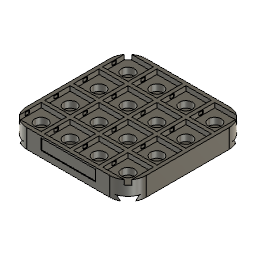
switchbox_choc (Autodesk Fusion 360 design; units mm, degrees)
Autodesk Fusion 360 part; units mm, degrees
sketch "outer_profile" plane through (0, 0, 0) normal (0, 0, 1) x (1, 0, 0)
  line L0 (32.8, 32.8) -> (-32.8, 32.8)
  line L1 (-32.8, 32.8) -> (-32.8, -32.8)
  line L2 (-32.8, -32.8) -> (32.8, -32.8)
  line L3 (32.8, -32.8) -> (32.8, 32.8)
  line L4 (-32.8, -32.8) -> (32.8, 32.8) construction
  dimension "d27" = 65.6
  dimension "d28" = 65.6
  constraint horizontal L0
  constraint horizontal L2
  constraint vertical L1
  constraint vertical L3
  constraint midpoint origin L4
  measures "d27" horizontal distance of L0.start L0.end
  measures "d28" vertical distance of L0.end L1.end
extrude "block" add sketch "outer_profile" along normal blind 10.45
fillet "corner_fillets" radius 10 4 edges at (32.8, -32.8, 5.225) (-32.8, -32.8, 5.225) (-32.8, 32.8, 5.225) (32.8, 32.8, 5.225)
ref_plane "WorkPlane1" through (0, 0, 10.45) normal (0, 0, 1) x (1, 0, 0)
sketch "pocket_seed" plane through (0, 0, 10.45) normal (0, 0, 1) x (1, 0, 0)
  line L0 (-16.9, -16.9) -> (-30.8, -16.9)
  line L1 (-30.8, -16.9) -> (-30.8, -30.8)
  line L2 (-30.8, -30.8) -> (-16.9, -30.8)
  line L3 (-16.9, -30.8) -> (-16.9, -16.9)
  line L4 (-30.8, -30.8) -> (-16.9, -16.9) construction
  dimension "d35" = 13.9
  dimension "d36" = 13.9
  dimension "d58" = 30.8
  dimension "d59" = 30.8
  constraint horizontal L0
  constraint horizontal L2
  constraint vertical L1
  constraint vertical L3
  measures "d35" horizontal distance of L0.start L0.end
  measures "d36" vertical distance of L0.end L1.end
  measures "d58" horizontal distance of origin L1.end
  measures "d59" vertical distance of origin L1.end
extrude "pocket_cut" cut sketch "pocket_seed" against normal blind 2.6
ref_plane "WorkPlane2" through (0, 0, 7.85) normal (0, 0, 1) x (1, 0, 0)
sketch "relief_seed" plane through (0, 0, 7.85) normal (0, 0, 1) x (1, 0, 0)
  circle A0 centre (-23.85, -23.85) radius 3.5
  dimension "d41" = 7
  dimension "d62" = 23.85
  dimension "d63" = 23.85
  measures "d41" diameter of A0
  measures "d62" horizontal distance of origin A0.centre
  measures "d63" vertical distance of origin A0.centre
extrude "relief_cut" cut sketch "relief_seed" against normal blind 3.6
ref_plane "WorkPlane3" through (0, 0, 8.45) normal (0, 0, 1) x (1, 0, 0)
sketch "rib_seed" plane through (0, 0, 8.45) normal (0, 0, 1) x (1, 0, 0)
  line L0 (-30.8, -25.6869) -> (-30.6, -23.85)
  line L1 (-30.6, -23.85) -> (-30.8, -23.2869)
  line L2 (-30.8, -23.2869) -> (-30.8, -25.6869)
  line L3 (-16.9, -24.6706) -> (-17.1, -23.85)
  line L4 (-17.1, -23.85) -> (-16.9, -22.2706)
  line L5 (-16.9, -22.2706) -> (-16.9, -24.6706)
  dimension "d91" = 30.8
  dimension "d92" = 30.6
  dimension "d93" = 2.4
  dimension "d94" = 23.85
  dimension "d95" = 16.9
  dimension "d96" = 17.1
  dimension "d97" = 2.4
  constraint vertical L2
  constraint vertical L5
  constraint horizontal L0.end L3.end
  measures "d91" horizontal distance of origin L0.start
  measures "d92" horizontal distance of origin L0.end
  measures "d93" vertical distance of L0.start L1.end
  measures "d94" vertical distance of origin L0.end
  measures "d95" horizontal distance of origin L3.start
  measures "d96" horizontal distance of origin L3.end
  measures "d97" vertical distance of L3.start L4.end
extrude "snap_ribs" add sketch "rib_seed" along normal blind 1.6
pattern_linear "pocket_grid" count 4 spacing 15.9 along (1, 0, 0) count 4 spacing 15.9 along (0, 1, 0) of "pocket_cut", "relief_cut", "snap_ribs"
sketch "stack_ring" plane through (0, 0, 0) normal (0, 0, 1) x (1, 0, 0)
  line L0 (31.6, 31.6) -> (-31.6, 31.6)
  line L1 (-31.6, 31.6) -> (-31.6, -31.6)
  line L2 (-31.6, -31.6) -> (31.6, -31.6)
  line L3 (31.6, -31.6) -> (31.6, 31.6)
  line L4 (-31.6, -31.6) -> (31.6, 31.6) construction
  dimension "d104" = 63.2
  dimension "d105" = 63.2
  constraint horizontal L0
  constraint horizontal L2
  constraint vertical L1
  constraint vertical L3
  constraint midpoint origin L4
  measures "d104" horizontal distance of L0.start L0.end
  measures "d105" vertical distance of L0.end L1.end
extrude "stack_ring_cut" cut sketch "stack_ring" along normal blind 2.5 draft 15
sketch "label_pocket" plane through (0, -32.8, 0) normal (0, -1, 0) x (1, 0, 0)
  line L0 (-22.8, 10.45) -> (-22.8, 0)
  line L1 (-22.8, 0) -> (22.8, 0)
  line L2 (22.8, 0) -> (22.8, 10.45)
  line L3 (22.8, 10.45) -> (-22.8, 10.45)
  line L4 (15, 9.45) -> (-15, 9.45)
  line L5 (-15, 9.45) -> (-15, 3.5)
  line L6 (-15, 3.5) -> (15, 3.5)
  line L7 (15, 3.5) -> (15, 9.45)
  line L8 (-15, 3.5) -> (15, 9.45) construction
  point P0 (0, 6.475)
  dimension "d123" = 30
  dimension "d124" = 5.95
  dimension "d125" = 6.475
  dimension "d126" = 0
  constraint midpoint L8 P0
  measures "d123" horizontal distance of L4.start L4.end
  measures "d124" vertical distance of L4.end L5.end
  measures "d125" vertical distance of origin P0
  measures "d126" horizontal distance of origin P0
extrude "label_cut" cut sketch "label_pocket" against normal blind 0.4 contours L4 L5 L6 L7
equation "cols = 4 mm" comment "Number of switch columns (2-10)"
equation "rows = 4 mm" comment "Number of switch rows (2-10)"
equation "wall = 2.0 mm" comment "Wall thickness in mm (min 1.75)"
equation "rib_depth = 0.2 mm" comment "Snap tightness in mm: lower is looser, 0.2 default"
equation "corner_fillet = 10 mm" comment "Vertical corner radius in mm"
equation "label_w = 30 mm" comment "Front label width in mm (auto-clamped to fit)"
equation "label_h = 12 mm" comment "Front label height in mm (auto-clamped to fit)"
equation "label_depth = 0.4 mm" comment "Front label recess depth in mm (auto-clamped)"
equation "stack_angle = 75 deg" comment "Stacking ring draft angle in degrees"
equation "pocket_size = 13.9 mm" comment "Switch pocket size (Choc)"
equation "pocket_depth = 2.6 mm" comment "Pocket depth to floor (Choc)"
equation "relief_dia = 7.0 mm" comment "Pin relief diameter"
equation "relief_depth = 3.6 mm" comment "Pin relief depth"
equation "floor_t = 1.75 mm" comment "Floor thickness below relief"
equation "ring_h = 2.5 mm" comment "Stack ring height"
equation "ring_inset = 1.2 mm" comment "Stack ring inset from outer wall"
equation "pitch = pocket_size + wall" comment "Pocket centre-to-centre pitch"
equation "box_x = ( cols / 1 mm ) * pitch + wall" comment "Overall box X"
equation "box_y = ( rows / 1 mm ) * pitch + wall" comment "Overall box Y"
equation "box_h = pocket_depth + relief_depth + floor_t + ring_h" comment "Overall box height"
equation "d27 = box_x"
equation "d28 = box_y"
equation "d29 = box_h"
equation "d32 = corner_fillet"
equation "d33 = box_h"
equation "d35 = pocket_size"
equation "d36 = pocket_size"
equation "d37 = -pocket_depth"
equation "d39 = box_h - pocket_depth"
equation "d41 = relief_dia"
equation "d42 = -relief_depth"
equation "rib_w = 2.4 mm" comment "Snap rib width along the pocket wall"
equation "rib_h = 1.6 mm" comment "Snap rib vertical height"
equation "rib_top_off = 0.4 mm" comment "Rib top offset below pocket mouth"
equation "d47 = box_h - rib_top_off - rib_h"
equation "seed_x = -( ( cols / 1 mm ) - 1 ) * pitch / 2" comment "Seed pocket centre X"
equation "seed_y = -( ( rows / 1 mm ) - 1 ) * pitch / 2" comment "Seed pocket centre Y"
equation "d58 = abs(seed_x) + pocket_size / 2"
equation "d59 = abs(seed_y) + pocket_size / 2"
equation "d62 = abs(seed_x)"
equation "d63 = abs(seed_y)"
equation "rib_wall_l = abs(seed_x) + pocket_size / 2" comment "Distance origin to left pocket wall"
equation "rib_wall_r = abs(seed_x) - pocket_size / 2" comment "Distance origin to right pocket wall"
equation "rib_tip_l = abs(seed_x) + pocket_size / 2 - rib_depth" comment "Left rib tip distance"
equation "rib_tip_r = abs(seed_x) - pocket_size / 2 + rib_depth" comment "Right rib tip distance"
equation "d91 = rib_wall_l"
equation "d92 = rib_tip_l"
equation "d93 = rib_w"
equation "d94 = abs(seed_y)"
equation "d95 = rib_wall_r"
equation "d96 = rib_tip_r"
equation "d97 = rib_w"
equation "d98 = rib_h"
equation "d100 = cols / 1 mm"
equation "d101 = rows / 1 mm"
equation "d102 = pitch"
equation "d103 = pitch"
equation "d104 = box_x - 2 * ring_inset"
equation "d105 = box_y - 2 * ring_inset"
equation "d106 = ring_h"
equation "d107 = 90 deg - stack_angle"
equation "label_w_max = box_x - 2 * corner_fillet - 2 mm" comment "Max label width for this box"
equation "label_w_eff = min(label_w; label_w_max)" comment "Effective label width (clamped)"
equation "label_band = box_h - ring_h - 2 mm" comment "Usable front-face height for the label"
equation "label_h_eff = min(label_h; label_band)" comment "Effective label height (clamped)"
equation "label_cz = ring_h + ( box_h - ring_h ) / 2" comment "Label centre height above bottom"
equation "label_d_eff = max(0.2 mm; min(label_depth; min(0.6 mm; wall - 1.2 mm)))" comment "Effective label depth: >=0.2mm, <=0.6mm, always leaving 1.2mm of wall"
equation "label_standoff = 1 mm" comment "Sketch plane offset outside the front face"
equation "d123 = label_w_eff"
equation "d124 = label_h_eff"
equation "d125 = label_cz"
equation "d127 = -( label_d_eff )"
named bodies: "box"
